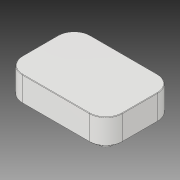
# Autodesk Inventor part: OM5P-AC
Saved by Autodesk Inventor 2018 (Build 220112000, 112)
## iProperties
Category: Loose
Company: Autodesk Inc.
Created: 2017-12-12
Part Number: OM5P-AC
Material: Generic
Document SubType Name: Modeling
Designer: Autodesk Inc.
Density: 1 g/cm^3
Appearance: Default
Catalog Web Link: http://www.open-mesh.ca/product/om5p-ac-dual-band-1-17-gbps-access-point/
Vendor: Andy Mark Inc.
Author: Autodesk Inc.
Keywords: Black Tote
Autodesk Inventor part; units mm, degrees
ref_plane "YZ Plane" through (0, 0, 0) normal (1, 0, 0) x (0, 1, 0)
sketch "Sketch1" plane through (0, 0, 0) normal (0, 1, 0) x (-1, 0, 0)
  line L0 (0, 0) -> (110, 0)
  line L1 (110, 0) -> (110, -75)
  line L2 (110, -75) -> (0, -75)
  line L3 (0, -75) -> (0, 0)
  dimension "d0" = 110
  dimension "d1" = 75
  constraints: 8 end point, 2 parallel, 1 horizontal, 1 perpendicular
  measures "d0" distance of L1.end L2.end
  measures "d1" distance of L0.end L1.end
extrude "Extrusion1" add sketch "Sketch1" along normal blind 27.5
fillet "Fillet1" radius 18 4 edges at (-110, 13.75, 0) (0, 13.75, 0) (0, 13.75, -75) (-110, 13.75, -75)
sketch "Sketch2" plane through (0, 0, 0) normal (0, -1, 0) x (1, 0, 0)
  line L0 (-110.0023, 0) -> (-0.0023, 0) construction
  line L1 (-0.0023, 0) -> (-0.0023, -81.8008) construction
  line L2 (-0.0023, -81.8008) -> (-110.0023, -81.8008) construction
  line L3 (-110.0023, -81.8008) -> (-110.0023, 0) construction
  arc A0 (-92, 0) -> (-110, -18) centre (-92, -18) ccw projected
  line L4 (-110.0023, 0) -> (-92, -18)
  circle A1 centre (-98.8278, -11.1731) radius 6.8778
  point P0 (0, 0)
  dimension "d14" = 110
  constraints: 2 end point, 1 centre point, 2 other
  measures "d14" distance of L0.start L0.end
extrude "Extrusion2" add sketch "Sketch2" along normal blind 2
sketch "Sketch3" plane through (-98.8278, -2, -11.1731) normal (0, -1, 0) x (1, 0, 0)
  circle A0 centre (0, 0) radius 6.25
  point P0 (98.8278, 11.1731)
  dimension "d28" = 12.5
  constraints: 1 centre point
  measures "d28" diameter of A0
extrude "Extrusion3" add sketch "Sketch3" along normal blind 0.5
ref_plane "Work Plane1" through (-92, 0, -37.5) normal (0, 0, 1) x (1, 0, 0)
ref_plane "Work Plane2" through (-55, 0, -18) normal (1, 0, 0) x (0, 0, -1)
mirror "Mirror1" about plane through (-92, 0, -37.5) normal (0, 0, 1) of "Extrusion2", "Extrusion3"
mirror "Mirror2" about plane through (-55, 0, -18) normal (1, 0, 0) of "Extrusion2", "Extrusion3", "Mirror1"
fillet "Fillet2" radius 0.5 16 edges at (-5.2721, 27.5, -5.2721) (0, 27.5, -37.5) (-5.2721, 27.5, -69.7279) (-55, 27.5, -75) (-104.7279, 27.5, -69.7279) (-110, 27.5, -37.5) (-104.7279, 27.5, -5.2721) (-55, 27.5, 0) (-104.7279, 0, -5.2721) (-110, 0, -37.5) (-104.7279, 0, -69.7279) (-55, 0, -75) (-5.2721, 0, -69.7279) (0, 0, -37.5) (-5.2721, 0, -5.2721) (-55, 0, 0)
body "Solid1"
